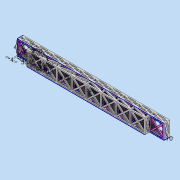
# Autodesk Inventor part: hashi1shado
Saved by Autodesk Inventor 2022 (Build 260153000, 153)
## iProperties
Created: 2024-05-14
Part Number: hashi1shado
Material: 一般
Document SubType Name: Modeling
Designer: ktamu
Density: 1 g/cm^3
Appearance: 既定
Mass: 103.699 g
Surface Area: 968.983 cm^2
Volume: 103.699 cm^3
Author: ktamu
Autodesk Inventor part; units mm, degrees
(part 1 of 2)
ref_plane "YZ Plane" through (0, 0, 0) normal (1, 0, 0) x (0, 1, 0)
ref_plane "XZ Plane" through (0, 0, 0) normal (0, 1, 0) x (-1, 0, 0)
ref_plane "XY Plane" through (0, 0, 0) normal (0, 0, 1) x (1, 0, 0)
sketch "スケッチ2" plane through (0, 0, 0) normal (1, 0, 0) x (0, 1, 0)
  line L0 (25, 10) -> (-25, 10)
  line L1 (-25, 10) -> (-25, -10)
  line L2 (-25, -10) -> (25, -10)
  line L3 (25, -10) -> (25, 10)
  line L4 (25, 10) -> (-25, -10) construction
  line L5 (-25, 10) -> (25, -10) construction
  point P0 (0, 0)
  dimension "d4" = 50
  dimension "d5" = 20
  constraints: 12 end point, 2 midpoint, 2 parallel, 1 horizontal, 1 perpendicular
  measures "d4" distance of L2.end L1.end
  measures "d5" distance of L1.end L0.end
sketch "スケッチ2 outline for 押し出し2" plane through (0, 0, 0) normal (1, 0, 0) x (0, 1, 0)
  line L0 (25, 10) -> (-25, 10)
  line L1 (25, -10) -> (25, 10)
  line L2 (-25, -10) -> (25, -10)
  line L3 (-25, 10) -> (-25, -10)
extrude "押し出し2" add sketch "スケッチ2 outline for 押し出し2" along normal mid plane 500
sketch "スケッチ3" plane through (-250, -25, 10) normal (0, 0, 1) x (1, 0, 0)
  circle A0 centre (250, 25) radius 5
  dimension "d8" = 10
  constraints: 1 centre point, 1 coincident
  measures "d8" diameter of A0
sketch "スケッチ3 outline for 押し出し3" plane through (-250, -25, 10) normal (0, 0, 1) x (1, 0, 0)
  circle A0 centre (250, 25) radius 5
extrude "押し出し3" add sketch "スケッチ3 outline for 押し出し3" along normal blind 2
sketch "SCfront" plane through (-250, -25, 10) normal (0, -1, 0) x (1, 0, 0)
  line L0 (0, -20) -> (500, -20)
  line L1 (500, 0) -> (500, -20)
  line L2 (500, 0) -> (0, 0)
  line L3 (0, -20) -> (0, 0)
  line L4 (0, 0) -> (500, 0)
  line L5 (500, 0) -> (500, -20)
  line L6 (500, -20) -> (0, -20)
  line L7 (0, -20) -> (0, 0)
  line L8 (0, 0) -> (500, -20) construction
  line L9 (500, 0) -> (0, -20) construction
  line L10 (0, 0) -> (500, 0)
  line L11 (0, -20) -> (500, -20)
  line L12 (0, 0) -> (50, 0)
  line L13 (50, 0) -> (50, -20)
  line L14 (50, -20) -> (0, -20)
  line L15 (0, -20) -> (0, 0)
  line L16 (100, 0) -> (100, -20)
  line L17 (150, 0) -> (150, -20)
  line L18 (200, 0) -> (200, -20)
  line L19 (250, 0) -> (250, -20)
  line L20 (450, 0) -> (450, -20)
  line L21 (400, 0) -> (400, -20)
  line L22 (350, 0) -> (350, -20)
  line L23 (300, 0) -> (300, -20)
  line L24 (0, 0) -> (0, -20)
  line L25 (0, 0) -> (50, -20)
  line L26 (0, -20) -> (50, 0) construction
  line L27 (50, 0) -> (100, -20)
  line L28 (100, 0) -> (50, -20)
  line L29 (52, -4) -> (98, -4)
  line L30 (98, -4) -> (98, -16)
  line L31 (98, -16) -> (52, -16)
  line L32 (52, -16) -> (52, -4)
  line L33 (75, -10) -> (98, -16) construction
  line L34 (98, -4) -> (52, -16) construction
  line L35 (102, -4) -> (148, -4)
  line L36 (102, -16) -> (102, -4)
  line L37 (148, -16) -> (102, -16)
  line L38 (148, -4) -> (148, -16)
  line L39 (152, -4) -> (198, -4)
  line L40 (152, -16) -> (152, -4)
  line L41 (198, -16) -> (152, -16)
  line L42 (198, -4) -> (198, -16)
  line L43 (202, -4) -> (248, -4)
  line L44 (202, -16) -> (202, -4)
  line L45 (248, -16) -> (202, -16)
  line L46 (248, -4) -> (248, -16)
  line L47 (252, -4) -> (298, -4)
  line L48 (252, -16) -> (252, -4)
  line L49 (298, -16) -> (252, -16)
  line L50 (298, -4) -> (298, -16)
  line L51 (302, -4) -> (348, -4)
  line L52 (302, -16) -> (302, -4)
  line L53 (348, -16) -> (302, -16)
  line L54 (348, -4) -> (348, -16)
  line L55 (352, -4) -> (398, -4)
  line L56 (352, -16) -> (352, -4)
  line L57 (398, -16) -> (352, -16)
  line L58 (398, -4) -> (398, -16)
  line L59 (402, -4) -> (448, -4)
  line L60 (402, -16) -> (402, -4)
  line L61 (448, -16) -> (402, -16)
  line L62 (448, -4) -> (448, -16)
  line L63 (48, -4) -> (48, -16)
  line L64 (48, -4) -> (4, -4)
  line L65 (4, -4) -> (4, -16.342138)
  line L66 (4, -16.342138) -> (48, -16.342138)
  line L67 (48, -16.342138) -> (48, -4)
  line L68 (452, -4) -> (452, -16)
  line L69 (452, -4) -> (496, -4)
  line L70 (496, -4) -> (496, -16.342138)
  line L71 (496, -16.342138) -> (452, -16.342138)
  line L72 (11.405237, -4) -> (48, -14.264946)
  line L73 (4, -6.077192) -> (40.594763, -16.342138)
  line L74 (488.594763, -4) -> (452, -14.264946)
  line L75 (496, -6.077192) -> (459.405237, -16.342138)
  line L76 (52, -4) -> (75, -10)
  line L77 (52, -6.066933) -> (90.076757, -16)
  line L78 (52.504844, -2.064765) -> (52.665247, -2.10661)
  line L79 (59.923243, -4) -> (98, -13.933067)
  line L80 (109.923243, -4) -> (148, -13.933067)
  line L81 (102, -6.066933) -> (140.076757, -16)
  line L82 (159.923243, -4) -> (198, -13.933067)
  line L83 (152, -6.066933) -> (190.076757, -16)
  line L84 (209.923243, -4) -> (248, -13.933067)
  line L85 (202, -6.066933) -> (240.076757, -16)
  line L86 (448, -6.066933) -> (409.923243, -16)
  line L87 (440.076757, -4) -> (402, -13.933067)
  line L88 (390.076757, -4) -> (352, -13.933067)
  line L89 (398, -6.066933) -> (359.923243, -16)
  line L90 (340.076757, -4) -> (302, -13.933067)
  line L91 (348, -6.066933) -> (309.923243, -16)
  line L92 (290.076757, -4) -> (252, -13.933067)
  line L93 (298, -6.066933) -> (259.923243, -16)
  line L94 (0, -10) -> (496, -10) construction
  line L95 (0, -10) -> (496, -10) construction
  line L96 (11.405237, -16) -> (48, -5.735054)
  line L97 (4, -13.922808) -> (39.375032, -4)
  line L98 (488.594763, -16) -> (452, -5.735054)
  line L99 (496, -13.922808) -> (459.405237, -3.657862)
  line L100 (52, -13.933067) -> (90.076757, -4)
  line L101 (59.923243, -16) -> (98, -6.066933)
  line L102 (109.923243, -16) -> (148, -6.066933)
  line L103 (102, -13.933067) -> (140.076757, -4)
  line L104 (159.923243, -16) -> (198, -6.066933)
  line L105 (152, -13.933067) -> (190.076757, -4)
  line L106 (209.923243, -16) -> (248, -6.066933)
  line L107 (202, -13.933067) -> (240.076757, -4)
  line L108 (448, -13.933067) -> (409.923243, -4)
  line L109 (440.076757, -16) -> (402, -6.066933)
  line L110 (398, -13.933067) -> (359.923243, -4)
  line L111 (390.076757, -16) -> (352, -6.066933)
  line L112 (348, -13.933067) -> (309.923243, -4)
  line L113 (340.076757, -16) -> (302, -6.066933)
  line L114 (298, -13.933067) -> (259.923243, -4)
  line L115 (290.076757, -16) -> (252, -6.066933)
  line L116 (25.390135, -12.077192) -> (10.185507, -16.342138)
  line L117 (474.609865, -12.077192) -> (489.814493, -16.342138)
  line L118 (50, 16) -> (50, -4)
  line L119 (100, 16) -> (100, -4)
  line L120 (150, 16) -> (150, -4)
  line L121 (250, 16) -> (250, -4)
  line L122 (450, 16) -> (450, -4)
  line L123 (300, 16) -> (300, -4)
  line L124 (350, 16) -> (350, -4)
  line L125 (400, 16) -> (400, -4)
  line L126 (200, 16) -> (200, -4)
  line L127 (152, 12) -> (198, 12)
  line L128 (198, 0) -> (152, 0)
  line L129 (152, 0) -> (152, 12)
  line L130 (148, 12) -> (148, 0)
  line L131 (109.923243, 12) -> (148, 2.066933)
  line L132 (148, 0) -> (102, 0)
  line L133 (102, 9.933067) -> (140.076757, 0)
  line L134 (102, 0) -> (102, 12)
  line L135 (50, 16) -> (100, -4)
  line L136 (100, 16) -> (50, -4)
  line L137 (102, 12) -> (148, 12)
  line L138 (52, 12) -> (98, 12)
  line L139 (98, 12) -> (98, 0)
  line L140 (98, 0) -> (52, 0)
  line L141 (52, 0) -> (52, 12)
  line L142 (75, 6) -> (98, 0) construction
  line L143 (98, 12) -> (52, 0) construction
  line L144 (198, 12) -> (198, 0)
  line L145 (202, 0) -> (202, 12)
  line L146 (248, 0) -> (202, 0)
  line L147 (248, 12) -> (248, 0)
  line L148 (202, 12) -> (248, 12)
  line L149 (252, 12) -> (298, 12)
  line L150 (59.923243, 12) -> (98, 2.066933)
  line L151 (59.923243, 0) -> (98, 9.933067)
  line L152 (52, 2.066933) -> (90.076757, 12)
  line L153 (52, 9.933067) -> (90.076757, 0)
  line L154 (352, 12) -> (398, 12)
  line L155 (352, 0) -> (352, 12)
  line L156 (398, 0) -> (352, 0)
  line L157 (398, 12) -> (398, 0)
  line L158 (402, 0) -> (402, 12)
  line L159 (402, 12) -> (448, 12)
  line L160 (448, 0) -> (402, 0)
  line L161 (448, 12) -> (448, 0)
  line L162 (52, 12) -> (75, 6)
  line L163 (252, 0) -> (252, 12)
  line L164 (298, 0) -> (252, 0)
  line L165 (298, 12) -> (298, 0)
  line L166 (302, 0) -> (302, 12)
  line L167 (302, 12) -> (348, 12)
  line L168 (348, 0) -> (302, 0)
  line L169 (348, 12) -> (348, 0)
  line L170 (52.504844, 13.935235) -> (52.665247, 13.89339)
  line L171 (209.923243, 12) -> (248, 2.066933)
  line L172 (202, 9.933067) -> (240.076757, 0)
  line L173 (209.923243, 0) -> (248, 9.933067)
  line L174 (202, 2.066933) -> (240.076757, 12)
  line L175 (448, 9.933067) -> (409.923243, 0)
  line L176 (440.076757, 12) -> (402, 2.066933)
  line L177 (448, 2.066933) -> (409.923243, 12)
  line L178 (440.076757, 0) -> (402, 9.933067)
  line L179 (290.076757, 12) -> (252, 2.066933)
  line L180 (290.076757, 0) -> (252, 9.933067)
  line L181 (298, 9.933067) -> (259.923243, 0)
  line L182 (298, 2.066933) -> (259.923243, 12)
  line L183 (340.076757, 12) -> (302, 2.066933)
  line L184 (340.076757, 0) -> (302, 9.933067)
  line L185 (348, 9.933067) -> (309.923243, 0)
  line L186 (348, 2.066933) -> (309.923243, 12)
  line L187 (398, 2.066933) -> (359.923243, 12)
  line L188 (390.076757, 12) -> (352, 2.066933)
  line L189 (390.076757, 0) -> (352, 9.933067)
  line L190 (398, 9.933067) -> (359.923243, 0)
  line L191 (102, 2.066933) -> (140.076757, 12)
  line L192 (109.923243, 0) -> (148, 9.933067)
  line L193 (152, 2.066933) -> (190.076757, 12)
  line L194 (159.923243, 12) -> (198, 2.066933)
  line L195 (159.923243, 0) -> (198, 9.933067)
  line L196 (152, 9.933067) -> (190.076757, 0)
  line L197 (50, 16) -> (450, 16)
  point P0 (250, -10)
  point P1 (440.076757, -4)
  point P2 (390.076757, -4)
  point P3 (340.076757, -4)
  point P4 (290.076757, -4)
  point P5 (209.923243, -4)
  point P6 (159.923243, -4)
  point P7 (109.923243, -4)
  point P8 (60.14392, -4.057568)
  point P9 (60, -4)
  point P10 (90, -16)
  point P11 (89.85608, -15.942432)
  point P12 (48, -14.264946)
  point P13 (40.594763, -3.657862)
  point P14 (482.015103, -10)
  point P15 (474.609865, -7.922808)
  point P16 (460.624968, -4)
  point P17 (467.204628, -10)
  point P18 (432.923243, -10)
  point P19 (425, -12.066933)
  point P20 (425, -7.933067)
  point P21 (417.076757, -10)
  point P22 (382.923243, -10)
  point P23 (375, -12.066933)
  point P24 (375, -7.933067)
  point P25 (367.076757, -10)
  point P26 (332.923243, -10)
  point P27 (325, -12.066933)
  point P28 (325, -7.933067)
  point P29 (317.076757, -10)
  point P30 (282.923243, -10)
  point P31 (275, -12.066933)
  point P32 (275, -7.933067)
  point P33 (267.076757, -10)
  point P34 (232.923243, -10)
  point P35 (225, -7.933067)
  point P36 (225, -12.066933)
  point P37 (217.076757, -10)
  point P38 (182.923243, -10)
  point P39 (175, -7.933067)
  point P40 (175, -12.066933)
  point P41 (167.076757, -10)
  point P42 (132.923243, -10)
  point P43 (125, -7.933067)
  point P44 (125, -12.066933)
  point P45 (117.076757, -10)
  point P46 (67.076757, -10)
  point P47 (59.923243, -16)
  point P48 (75, -12.066933)
  point P49 (75, -7.933067)
  point P50 (82.923243, -10)
  point P51 (25.390135, -7.922808)
  point P52 (32.795372, -10)
  point P53 (48, -5.735054)
  point P54 (11.405237, -16)
  point P55 (17.984897, -10)
  point P56 (4, -13.922808)
  point P57 (250, 6)
  point P58 (89.85608, 0.057568)
  point P59 (75, 3.933067)
  point P60 (60.14392, 0.057568)
  point P61 (60, 0)
  point P62 (90, 0)
  point P63 (67.076757, 6)
  point P64 (75, 8.066933)
  point P65 (89.85608, 11.942432)
  point P66 (90, 12)
  point P67 (60, 12)
  point P68 (60.14392, 11.942432)
  point P69 (82.923243, 6)
  point P70 (117.076757, 6)
  point P71 (125, 3.933067)
  point P72 (125, 8.066933)
  point P73 (109.923243, 12)
  point P74 (132.923243, 6)
  point P75 (148, 2.066933)
  point P76 (167.076757, 6)
  point P77 (159.923243, 12)
  point P78 (175, 8.066933)
  point P79 (175, 3.933067)
  point P80 (182.923243, 6)
  point P81 (198, 2.066933)
  point P82 (225, 3.933067)
  point P83 (217.076757, 6)
  point P84 (225, 8.066933)
  point P85 (209.923243, 12)
  point P86 (232.923243, 6)
  point P87 (248, 2.066933)
  point P88 (267.076757, 6)
  point P89 (252, 2.066933)
  point P90 (275, 3.933067)
  point P91 (275, 8.066933)
  point P92 (290.076757, 12)
  point P93 (282.923243, 6)
  point P94 (317.076757, 6)
  point P95 (302, 2.066933)
  point P96 (325, 3.933067)
  point P97 (325, 8.066933)
  point P98 (340.076757, 12)
  point P99 (332.923243, 6)
  point P100 (367.076757, 6)
  point P101 (352, 2.066933)
  point P102 (375, 8.066933)
  point P103 (390.076757, 12)
  point P104 (375, 3.933067)
  point P105 (382.923243, 6)
  point P106 (417.076757, 6)
  point P107 (402, 2.066933)
  point P108 (425, 3.933067)
  point P109 (425, 8.066933)
  point P110 (440.076757, 12)
  point P111 (432.923243, 6)
  point P112 (59.923243, 0)
  dimension "d12" = 50
  dimension "d15" = 50
  dimension "d20" = 46
  dimension "d21" = 12
  dimension "d24" = 50
  dimension "d29" = 4
  dimension "d30" = 4
  dimension "d33" = 4
  dimension "d37" = 2
  dimension "d40" = 50
  dimension "d96" = 0
  dimension "d97" = 10
  dimension "d106" = 16
  constraints: 382 end point, 73 symmetric about line, 28 horizontal alignment, 25 parallel, 25 point on line, 15 collinear, 8 midpoint, 7 horizontal, 5 perpendicular, 2 vertical, 228 other
  measures "d12" distance of L13.end L14.end
  measures "d15" distance of L12.end L16.start
  measures "d20" distance of L30.end L31.end
  measures "d21" distance of L29.end L30.end
  measures "d24" distance of L29.start L35.start
  measures "d29" distance between parallel lines of L32 L63
  measures "d30" distance between parallel lines of L65 L3
  measures "d33" distance between parallel lines of L12 L64
  measures "d37" distance between parallel lines of L76 L77
  measures "d40" distance of L79.start L80.start
  measures "d96" distance between parallel lines of L94 L95
  measures "d97" distance between parallel lines of L0 L95
  measures "d106" distance of L12.end L118.start
sketch "SCfront outline for 押し出し4" plane through (-250, -25, 10) normal (0, -1, 0) x (1, 0, 0)
  line L0 (496, -6.077192) -> (459.405237, -16.342138)
  line L1 (496, -16.342138) -> (496, -6.077192)
  line L2 (459.405237, -16.342138) -> (496, -16.342138)
  line L3 (452, -14.264946) -> (488.594763, -4)
  line L4 (452, -4) -> (452, -14.264946)
  line L5 (488.594763, -4) -> (452, -4)
  line L6 (448, -6.066933) -> (409.923243, -16)
  line L7 (448, -16) -> (448, -6.066933)
  line L8 (409.923243, -16) -> (448, -16)
  line L9 (402, -13.933067) -> (440.076757, -4)
  line L10 (402, -4) -> (402, -13.933067)
  line L11 (440.076757, -4) -> (402, -4)
  line L12 (398, -6.066933) -> (359.923243, -16)
  line L13 (398, -16) -> (398, -6.066933)
  line L14 (359.923243, -16) -> (398, -16)
  line L15 (352, -13.933067) -> (390.076757, -4)
  line L16 (352, -4) -> (352, -13.933067)
  line L17 (390.076757, -4) -> (352, -4)
  line L18 (348, -6.066933) -> (309.923243, -16)
  line L19 (348, -16) -> (348, -6.066933)
  line L20 (309.923243, -16) -> (348, -16)
  line L21 (302, -13.933067) -> (340.076757, -4)
  line L22 (302, -4) -> (302, -13.933067)
  line L23 (340.076757, -4) -> (302, -4)
  line L24 (298, -6.066933) -> (259.923243, -16)
  line L25 (298, -16) -> (298, -6.066933)
  line L26 (259.923243, -16) -> (298, -16)
  line L27 (252, -13.933067) -> (290.076757, -4)
  line L28 (252, -4) -> (252, -13.933067)
  line L29 (290.076757, -4) -> (252, -4)
  line L30 (209.923243, -4) -> (248, -13.933067)
  line L31 (248, -4) -> (209.923243, -4)
  line L32 (248, -13.933067) -> (248, -4)
  line L33 (240.076757, -16) -> (202, -6.066933)
  line L34 (202, -16) -> (240.076757, -16)
  line L35 (202, -6.066933) -> (202, -16)
  line L36 (159.923243, -4) -> (198, -13.933067)
  line L37 (198, -4) -> (159.923243, -4)
  line L38 (198, -13.933067) -> (198, -4)
  line L39 (190.076757, -16) -> (152, -6.066933)
  line L40 (152, -16) -> (190.076757, -16)
  line L41 (152, -6.066933) -> (152, -16)
  line L42 (109.923243, -4) -> (148, -13.933067)
  line L43 (148, -4) -> (109.923243, -4)
  line L44 (148, -13.933067) -> (148, -4)
  line L45 (140.076757, -16) -> (102, -6.066933)
  line L46 (102, -16) -> (140.076757, -16)
  line L47 (102, -6.066933) -> (102, -16)
  line L48 (60.14392, -4.057568) -> (98, -13.933067)
  line L49 (60, -4) -> (60.14392, -4.057568)
  line L50 (98, -4) -> (60, -4)
  line L51 (98, -13.933067) -> (98, -4)
  line L52 (89.85608, -15.942432) -> (52, -6.066933)
  line L53 (90, -16) -> (89.85608, -15.942432)
  line L54 (52, -16) -> (90, -16)
  line L55 (52, -6.066933) -> (52, -16)
  line L56 (11.405237, -4) -> (48, -14.264946)
  line L57 (48, -4) -> (11.405237, -4)
  line L58 (48, -14.264946) -> (48, -4)
  line L59 (40.594763, -16.342138) -> (4, -6.077192)
  line L60 (4, -16.342138) -> (40.594763, -16.342138)
  line L61 (4, -6.077192) -> (4, -16.342138)
extrude "押し出し4" cut sketch "SCfront outline for 押し出し4" against normal through all
sketch "SCLeft" plane through (-250, 0, 0) normal (-1, 0, 0) x (0, 0, 1)
  line L0 (10, 25) -> (10, -25)
  line L1 (-10, 25) -> (10, 25)
  line L2 (10, 25) -> (10, -25)
  line L3 (10, -25) -> (-10, -25)
  line L4 (-10, -25) -> (-10, 25)
  line L5 (-10, 25) -> (10, -25) construction
  line L6 (10, 25) -> (-10, -25) construction
  line L7 (-6, 21) -> (6, 21)
  line L8 (6, 21) -> (6, -21)
  line L9 (6, -21) -> (-6, -21)
  line L10 (-6, -21) -> (-6, 21)
  line L11 (-6, 21) -> (-1.040016, 3.640055) construction
  line L12 (6, 21) -> (-6, -21) construction
  line L13 (7.415352, 0) -> (4.34275, 0)
  line L14 (2.080031, 0) -> (6, -13.71989)
  line L15 (-3.919969, 21) -> (0, 7.28011)
  line L16 (-6, 21) -> (-1.040016, 3.640055)
  line L17 (1.040016, -3.640055) -> (6, -21)
  line L18 (-6, 13.71989) -> (-2.080031, 0)
  line L19 (0, -7.28011) -> (3.919969, -21)
  line L20 (0, 7.28011) -> (3.919969, 21)
  line L21 (-6, -13.71989) -> (-2.080031, 0)
  line L22 (-3.919969, -21) -> (0, -7.28011)
  line L23 (2.080031, 0) -> (6, 13.71989)
  point P0 (0, 0)
  dimension "d47" = 12
  dimension "d48" = 42
  constraints: 46 end point, 8 parallel, 5 point on line, 4 symmetric about line, 3 horizontal, 3 midpoint, 2 perpendicular
  measures "d47" distance of L8.end L9.end
  measures "d48" distance of L7.end L8.end
sketch "SCLeft outline for 押し出し5left" plane through (-250, 0, 0) normal (-1, 0, 0) x (0, 0, 1)
  line L0 (-6, 21) -> (-6, -21)
  line L1 (6, 21) -> (-6, 21)
  line L2 (6, -21) -> (6, 21)
  line L3 (-6, -21) -> (6, -21)
extrude "押し出し5left" cut sketch "SCLeft outline for 押し出し5left" against normal through all
sketch "SCLeft outline for 押し出し6" plane through (-250, 0, 0) normal (-1, 0, 0) x (0, 0, 1)
  line L0 (2.080031, 0) -> (6, 13.71989)
  line L1 (6, -13.71989) -> (2.080031, 0)
  line L2 (6, -21) -> (6, -13.71989)
  line L3 (3.919969, -21) -> (6, -21)
  line L4 (0, -7.28011) -> (3.919969, -21)
  line L5 (-3.919969, -21) -> (0, -7.28011)
  line L6 (-6, -21) -> (-3.919969, -21)
  line L7 (-6, -13.71989) -> (-6, -21)
  line L8 (-2.080031, 0) -> (-6, -13.71989)
  line L9 (-6, 13.71989) -> (-2.080031, 0)
  line L10 (-6, 21) -> (-6, 13.71989)
  line L11 (-3.919969, 21) -> (-6, 21)
  line L12 (0, 7.28011) -> (-3.919969, 21)
  line L13 (3.919969, 21) -> (0, 7.28011)
  line L14 (6, 21) -> (3.919969, 21)
  line L15 (6, 13.71989) -> (6, 21)
extrude "押し出し6" add sketch "SCLeft outline for 押し出し6" against normal blind 4
mirror "ミラー1" about plane through (0, 0, 0) normal (1, 0, 0) of "押し出し6"
sketch "SCtop" plane through (-250, -25, 10) normal (0, 0, 1) x (1, 0, 0)
  circle A0 centre (250, 25) radius 5
  line L0 (500, 0) -> (0, 0)
  line L1 (500, 50) -> (500, 0)
  line L2 (0, 50) -> (500, 50)
  line L3 (0, 0) -> (0, 50)
  circle A1 centre (250, 25) radius 5
  line L4 (0, 0) -> (0, 50)
  line L5 (0, 50) -> (500, 0) construction
  line L6 (0, 0) -> (500, 0)
  line L7 (500, 50) -> (0, 0) construction
  line L8 (0, 50) -> (500, 50)
  line L9 (500, 50) -> (500, 0)
  line L10 (500, 0) -> (0, 0)
  line L11 (0, 0) -> (0, 50)
  line L12 (0, 50) -> (500, 0) construction
  line L13 (500, 50) -> (0, 0) construction
  line L14 (0, 50) -> (500, 50)
  line L15 (0, 50) -> (50, 50)
  line L16 (50, 50) -> (50, 0)
  line L17 (50, 0) -> (0, 0)
  line L18 (0, 0) -> (0, 50)
  line L19 (100, 50) -> (100, 0)
  line L20 (150, 50) -> (150, 0)
  line L21 (200, 50) -> (200, 0)
  line L22 (250, 50) -> (250, 0)
  line L23 (300, 50) -> (300, 0)
  line L24 (350, 50) -> (350, 0)
  line L25 (400, 50) -> (400, 0)
  line L26 (450, 50) -> (450, 0)
  line L27 (50, 50) -> (100, 0)
  line L28 (0, 50) -> (50, 0)
  line L29 (50, 50) -> (0, 0)
  line L30 (98, 4) -> (60.14392, 4)
  line L31 (52, 46) -> (98, 46)
  line L32 (98, 46) -> (98, 4)
  line L33 (98, 4) -> (52, 4)
  line L34 (52, 4) -> (52, 46)
  line L35 (4, 46) -> (48, 46)
  line L36 (48, 46) -> (48, 4)
  line L37 (48, 4) -> (4, 4)
  line L38 (4, 4) -> (4, 46)
  line L39 (6.828427, 46) -> (48.025843, 4.802584)
  line L40 (4, 43.171573) -> (43.171573, 4)
  line L41 (25, 25) -> (25, 18.621886)
  line L42 (98, 0) -> (98, 4)
  line L43 (53.475936, 44.652406) -> (98, 4)
  line L44 (52, 43.291755) -> (95.033826, 4)
  line L45 (54.966174, 46) -> (98, 6.708245)
  line L46 (98, 43.291755) -> (54.966174, 4)
  line L47 (92.274678, 40.772532) -> (53.475936, 5.347594)
  line L48 (95.033826, 46) -> (52, 6.708245)
  line L49 (50.144939, 5.014494) -> (50, 4.882159)
  line L50 (73.584326, 23.584326) -> (90.909091, 40.909091)
  line L51 (92.274678, 40.772532) -> (73.516913, 23.645877) construction
  line L52 (53.475936, 5.347594) -> (52, 4) construction
  line L53 (52, 46) -> (53.475936, 44.652406) construction
  line L54 (73.516913, 26.354123) -> (98, 4) construction
  line L55 (48, 46) -> (4, 4)
  line L56 (45.103446, 46) -> (4, 6.764892)
  line L57 (48, 43.235108) -> (6.896554, 4)
  line L58 (104.966174, 46) -> (148, 6.708245)
  line L59 (145.033826, 46) -> (102, 6.708245)
  line L60 (148, 43.291755) -> (104.966174, 4)
  line L61 (102, 43.291755) -> (145.033826, 4)
  line L62 (148, 46) -> (148, 4)
  line L63 (102, 46) -> (148, 46)
  line L64 (102, 4) -> (102, 46)
  line L65 (148, 4) -> (102, 4)
  line L66 (154.966174, 46) -> (198, 6.708245)
  line L67 (195.033826, 46) -> (152, 6.708245)
  line L68 (198, 43.291755) -> (154.966174, 4)
  line L69 (152, 43.291755) -> (195.033826, 4)
  line L70 (198, 46) -> (198, 4)
  line L71 (152, 46) -> (198, 46)
  line L72 (152, 4) -> (152, 46)
  line L73 (198, 4) -> (152, 4)
  line L74 (204.966174, 46) -> (248, 6.708245)
  line L75 (245.033826, 46) -> (202, 6.708245)
  line L76 (248, 43.291755) -> (204.966174, 4)
  line L77 (202, 43.291755) -> (245.033826, 4)
  line L78 (248, 46) -> (248, 4)
  line L79 (202, 46) -> (248, 46)
  line L80 (202, 4) -> (202, 46)
  line L81 (248, 4) -> (202, 4)
  line L82 (254.966174, 46) -> (298, 6.708245)
  line L83 (295.033826, 46) -> (252, 6.708245)
  line L84 (298, 43.291755) -> (254.966174, 4)
  line L85 (252, 43.291755) -> (295.033826, 4)
  line L86 (298, 46) -> (298, 4)
  line L87 (252, 46) -> (298, 46)
  line L88 (252, 4) -> (252, 46)
  line L89 (298, 4) -> (252, 4)
  line L90 (304.966174, 46) -> (348, 6.708245)
  line L91 (345.033826, 46) -> (302, 6.708245)
  line L92 (348, 43.291755) -> (304.966174, 4)
  line L93 (302, 43.291755) -> (345.033826, 4)
  line L94 (348, 46) -> (348, 4)
  line L95 (302, 46) -> (348, 46)
  line L96 (302, 4) -> (302, 46)
  line L97 (348, 4) -> (302, 4)
  line L98 (354.966174, 46) -> (398, 6.708245)
  line L99 (395.033826, 46) -> (352, 6.708245)
  line L100 (398, 43.291755) -> (354.966174, 4)
  line L101 (352, 43.291755) -> (395.033826, 4)
  line L102 (398, 46) -> (398, 4)
  line L103 (352, 46) -> (398, 46)
  line L104 (352, 4) -> (352, 46)
  line L105 (398, 4) -> (352, 4)
  line L106 (404.966174, 46) -> (448, 6.708245)
  line L107 (445.033826, 46) -> (402, 6.708245)
  line L108 (448, 43.291755) -> (404.966174, 4)
  line L109 (402, 43.291755) -> (445.033826, 4)
  line L110 (448, 46) -> (448, 4)
  line L111 (402, 46) -> (448, 46)
  line L112 (402, 4) -> (402, 46)
  line L113 (448, 4) -> (402, 4)
  line L114 (496, 46) -> (452, 46)
  line L115 (452, 46) -> (452, 4)
  line L116 (452, 4) -> (496, 4)
  line L117 (496, 4) -> (496, 46)
  line L118 (493.171573, 46) -> (451.974157, 4.802584)
  line L119 (496, 43.171573) -> (456.828427, 4)
  line L120 (454.896554, 46) -> (496, 6.764892)
  line L121 (452, 43.235108) -> (493.103446, 4)
  point P0 (75, 25)
  point P1 (123.516913, 26.354123)
  point P2 (123.584326, 23.584326)
  point P3 (123.516913, 23.645877)
  point P4 (173.516913, 26.354123)
  point P5 (173.584326, 23.584326)
  point P6 (173.516913, 23.645877)
  point P7 (223.516913, 26.354123)
  point P8 (223.584326, 23.584326)
  point P9 (223.516913, 23.645877)
  point P10 (273.516913, 26.354123)
  point P11 (273.584326, 23.584326)
  point P12 (273.516913, 23.645877)
  point P13 (323.516913, 26.354123)
  point P14 (323.584326, 23.584326)
  point P15 (323.516913, 23.645877)
  point P16 (373.516913, 26.354123)
  point P17 (373.584326, 23.584326)
  point P18 (373.516913, 23.645877)
  point P19 (423.516913, 26.354123)
  point P20 (423.584326, 23.584326)
  point P21 (423.516913, 23.645877)
  point P22 (474.544134, 21.715707)
  point P23 (477.373326, 24.544899)
  point P24 (474.479122, 27.307549)
  point P25 (452, 4.828427)
  point P26 (471.64993, 24.478357)
  point P27 (427.966174, 25)
  point P28 (425, 22.291755)
  point P29 (425, 27.708245)
  point P30 (375, 22.291755)
  point P31 (375, 27.708245)
  point P32 (422.033826, 25)
  point P33 (377.966174, 25)
  point P34 (372.033826, 25)
  point P35 (327.966174, 25)
  point P36 (325, 22.291755)
  point P37 (325, 27.708245)
  point P38 (322.033826, 25)
  point P39 (275, 22.291755)
  point P40 (277.966174, 25)
  point P41 (275, 27.708245)
  point P42 (252, 20.417424)
  point P43 (272.033826, 25)
  point P44 (252, 29.582576)
  point P45 (225, 22.291755)
  point P46 (248, 29.582576)
  point P47 (227.966174, 25)
  point P48 (248, 20.417424)
  point P49 (225, 27.708245)
  point P50 (222.033826, 25)
  point P51 (175, 22.291755)
  point P52 (177.966174, 25)
  point P53 (175, 27.708245)
  point P54 (172.033826, 25)
  point P55 (125, 22.291755)
  point P56 (127.966174, 25)
  point P57 (125, 27.708245)
  point P58 (122.033826, 25)
  point P59 (77.966174, 25)
  point P60 (75, 22.291755)
  point P61 (75, 27.708245)
  point P62 (72.033826, 25)
  point P63 (25.455866, 21.715707)
  point P64 (28.35007, 24.478357)
  point P65 (48, 4.828427)
  point P66 (22.626674, 24.544899)
  point P67 (25.520878, 27.307549)
  dimension "d55" = 50
  dimension "d56" = 50
  dimension "d59" = 50
  dimension "d64" = 46
  dimension "d65" = 42
  dimension "d66" = 44
  dimension "d67" = 42
  dimension "d68" = 4
  dimension "d69" = 4
  dimension "d76" = 2
  dimension "d77" = 2
  dimension "d80" = 50
  constraints: 226 end point, 97 point on line, 20 midpoint, 17 parallel, 12 symmetric about line, 6 horizontal, 5 perpendicular, 1 vertical, 185 other
  measures "d55" distance of L16.end L17.end
  measures "d56" distance of L15.end L16.end
  measures "d59" distance of L15.end L19.start
  measures "d64" distance of L30.start L33.end
  measures "d65" distance of L31.end L30.start
  measures "d66" distance of L36.end L37.end
  measures "d67" distance of L35.end L36.end
  measures "d68" distance between parallel lines of L2 L35
  measures "d69" distance between parallel lines of L34 L36
  measures "d76" distance between parallel lines of L55 L56
  measures "d77" distance between parallel lines of L55 L57
  measures "d80" distance of L45.start L58.start
sketch "SCtop outline for 押し出し7" plane through (-250, -25, 10) normal (0, 0, 1) x (1, 0, 0)
  line L0 (456.828427, 4) -> (493.103446, 4)
  line L1 (474.544134, 21.715707) -> (456.828427, 4)
  line L2 (493.103446, 4) -> (474.544134, 21.715707)
  line L3 (496, 6.764892) -> (496, 43.171573)
  line L4 (477.373326, 24.544899) -> (496, 6.764892)
  line L5 (496, 43.171573) -> (477.373326, 24.544899)
  line L6 (493.171573, 46) -> (454.896554, 46)
  line L7 (474.479122, 27.307549) -> (493.171573, 46)
  line L8 (454.896554, 46) -> (474.479122, 27.307549)
  line L9 (452, 43.235108) -> (452, 4.828427)
  line L10 (471.64993, 24.478357) -> (452, 43.235108)
  line L11 (452, 4.828427) -> (471.64993, 24.478357)
  line L12 (448, 6.708245) -> (448, 43.291755)
  line L13 (427.966174, 25) -> (448, 6.708245)
  line L14 (448, 43.291755) -> (427.966174, 25)
  line L15 (404.966174, 4) -> (445.033826, 4)
  line L16 (425, 22.291755) -> (404.966174, 4)
  line L17 (445.033826, 4) -> (425, 22.291755)
  line L18 (445.033826, 46) -> (404.966174, 46)
  line L19 (425, 27.708245) -> (445.033826, 46)
  line L20 (404.966174, 46) -> (425, 27.708245)
  line L21 (354.966174, 4) -> (395.033826, 4)
  line L22 (375, 22.291755) -> (354.966174, 4)
  line L23 (395.033826, 4) -> (375, 22.291755)
  line L24 (395.033826, 46) -> (354.966174, 46)
  line L25 (375, 27.708245) -> (395.033826, 46)
  line L26 (354.966174, 46) -> (375, 27.708245)
  line L27 (402, 43.291755) -> (402, 6.708245)
  line L28 (422.033826, 25) -> (402, 43.291755)
  line L29 (402, 6.708245) -> (422.033826, 25)
  line L30 (398, 6.708245) -> (398, 43.291755)
  line L31 (377.966174, 25) -> (398, 6.708245)
  line L32 (398, 43.291755) -> (377.966174, 25)
  line L33 (352, 43.291755) -> (352, 6.708245)
  line L34 (372.033826, 25) -> (352, 43.291755)
  line L35 (352, 6.708245) -> (372.033826, 25)
  line L36 (348, 6.708245) -> (348, 43.291755)
  line L37 (327.966174, 25) -> (348, 6.708245)
  line L38 (348, 43.291755) -> (327.966174, 25)
  line L39 (304.966174, 4) -> (345.033826, 4)
  line L40 (325, 22.291755) -> (304.966174, 4)
  line L41 (345.033826, 4) -> (325, 22.291755)
  line L42 (345.033826, 46) -> (304.966174, 46)
  line L43 (325, 27.708245) -> (345.033826, 46)
  line L44 (304.966174, 46) -> (325, 27.708245)
  line L45 (302, 43.291755) -> (302, 6.708245)
  line L46 (322.033826, 25) -> (302, 43.291755)
  line L47 (302, 6.708245) -> (322.033826, 25)
  line L48 (254.966174, 4) -> (295.033826, 4)
  line L49 (275, 22.291755) -> (254.966174, 4)
  line L50 (295.033826, 4) -> (275, 22.291755)
  line L51 (298, 6.708245) -> (298, 43.291755)
  line L52 (277.966174, 25) -> (298, 6.708245)
  line L53 (298, 43.291755) -> (277.966174, 25)
  line L54 (295.033826, 46) -> (254.966174, 46)
  line L55 (275, 27.708245) -> (295.033826, 46)
  line L56 (254.966174, 46) -> (275, 27.708245)
  line L57 (252, 20.417424) -> (252, 6.708245)
  arc A0 (252, 29.582576) -> (252, 20.417424) centre (250, 25) cw
  line L58 (252, 43.291755) -> (252, 29.582576)
  line L59 (272.033826, 25) -> (252, 43.291755)
  line L60 (252, 6.708245) -> (272.033826, 25)
  line L61 (204.966174, 4) -> (245.033826, 4)
  line L62 (225, 22.291755) -> (204.966174, 4)
  line L63 (245.033826, 4) -> (225, 22.291755)
  line L64 (248, 29.582576) -> (248, 43.291755)
  arc A1 (248, 20.417424) -> (248, 29.582576) centre (250, 25) cw
  line L65 (248, 6.708245) -> (248, 20.417424)
  line L66 (227.966174, 25) -> (248, 6.708245)
  line L67 (248, 43.291755) -> (227.966174, 25)
  line L68 (245.033826, 46) -> (204.966174, 46)
  line L69 (225, 27.708245) -> (245.033826, 46)
  line L70 (204.966174, 46) -> (225, 27.708245)
  line L71 (202, 43.291755) -> (202, 6.708245)
  line L72 (222.033826, 25) -> (202, 43.291755)
  line L73 (202, 6.708245) -> (222.033826, 25)
  line L74 (154.966174, 4) -> (195.033826, 4)
  line L75 (175, 22.291755) -> (154.966174, 4)
  line L76 (195.033826, 4) -> (175, 22.291755)
  line L77 (198, 6.708245) -> (198, 43.291755)
  line L78 (177.966174, 25) -> (198, 6.708245)
  line L79 (198, 43.291755) -> (177.966174, 25)
  line L80 (195.033826, 46) -> (154.966174, 46)
  line L81 (175, 27.708245) -> (195.033826, 46)
  line L82 (154.966174, 46) -> (175, 27.708245)
  line L83 (152, 43.291755) -> (152, 6.708245)
  line L84 (172.033826, 25) -> (152, 43.291755)
  line L85 (152, 6.708245) -> (172.033826, 25)
  line L86 (104.966174, 4) -> (145.033826, 4)
  line L87 (125, 22.291755) -> (104.966174, 4)
  line L88 (145.033826, 4) -> (125, 22.291755)
  line L89 (148, 6.708245) -> (148, 43.291755)
  line L90 (127.966174, 25) -> (148, 6.708245)
  line L91 (148, 43.291755) -> (127.966174, 25)
  line L92 (145.033826, 46) -> (104.966174, 46)
  line L93 (125, 27.708245) -> (145.033826, 46)
  line L94 (104.966174, 46) -> (125, 27.708245)
  line L95 (102, 43.291755) -> (102, 6.708245)
  line L96 (122.033826, 25) -> (102, 43.291755)
  line L97 (102, 6.708245) -> (122.033826, 25)
  line L98 (98, 43.291755) -> (77.966174, 25)
  line L99 (98, 6.708245) -> (98, 43.291755)
  line L100 (77.966174, 25) -> (98, 6.708245)
  line L101 (75, 22.291755) -> (54.966174, 4)
  line L102 (54.966174, 4) -> (95.033826, 4)
  line L103 (95.033826, 4) -> (75, 22.291755)
  line L104 (75, 27.708245) -> (95.033826, 46)
  line L105 (54.966174, 46) -> (75, 27.708245)
  line L106 (95.033826, 46) -> (54.966174, 46)
  line L107 (52, 6.708245) -> (72.033826, 25)
  line L108 (52, 43.291755) -> (52, 6.708245)
  line L109 (72.033826, 25) -> (52, 43.291755)
  line L110 (25.455866, 21.715707) -> (6.896554, 4)
  line L111 (43.171573, 4) -> (25.455866, 21.715707)
  line L112 (6.896554, 4) -> (43.171573, 4)
  line L113 (48, 43.235108) -> (28.35007, 24.478357)
  line L114 (48, 4.828427) -> (48, 43.235108)
  line L115 (28.35007, 24.478357) -> (48, 4.828427)
  line L116 (4, 6.764892) -> (22.626674, 24.544899)
  line L117 (4, 43.171573) -> (4, 6.764892)
  line L118 (22.626674, 24.544899) -> (4, 43.171573)
  line L119 (25.520878, 27.307549) -> (45.103446, 46)
  line L120 (6.828427, 46) -> (25.520878, 27.307549)
  line L121 (45.103446, 46) -> (6.828427, 46)
extrude "押し出し7" cut sketch "SCtop outline for 押し出し7" against normal through all
sketch "スケッチ7" plane through (0, 0, 12) normal (0, 0, 1) x (1, 0, 0)
  line L0 (-2, 21) -> (-2, -21)
  line L1 (2, -18.291755) -> (2, -4.582576)
  line L2 (2, -21) -> (2, 21)
  circle A0 centre (0, 0) radius 5
  arc A1 (-2, -4.582576) -> (2, -4.582576) centre (0, 0) ccw
  line L3 (-2, -4.582576) -> (-2, 4.582576)
  line L4 (2, -4.582576) -> (2, 4.582576)
  circle A2 centre (0, 0) radius 1
  point P0 (-2, -4.582576)
  dimension "d89" = 2
  constraints: 4 end point, 2 point on circle, 2 point on line, 1 centre point, 1 coincident
  measures "d89" diameter of A2
sketch "スケッチ7 outline for 押し出し8" plane through (0, 0, 12) normal (0, 0, 1) x (1, 0, 0)
  arc A0 (2, -4.582576) -> (2, 4.582576) centre (0, 0) ccw
  line L0 (2, 4.582576) -> (2, -4.582576)
  arc A1 (-2, 4.582576) -> (-2, -4.582576) centre (0, 0) ccw
  line L1 (-2, -4.582576) -> (-2, 4.582576)
extrude "押し出し8" cut sketch "スケッチ7 outline for 押し出し8" against normal through all
sketch "スケッチ7 outline for 押し出し9" plane through (0, 0, 12) normal (0, 0, 1) x (1, 0, 0)
  arc A0 (-2, -4.582576) -> (2, -4.582576) centre (0, 0) ccw
  line L0 (-2, 4.582576) -> (-2, -4.582576)
  line L1 (2, -4.582576) -> (2, 4.582576)
  arc A1 (2, 4.582576) -> (-2, 4.582576) centre (0, 0) ccw
  circle A2 centre (0, 0) radius 1
extrude "押し出し9" cut sketch "スケッチ7 outline for 押し出し9" against normal blind 2
sketch "スケッチ7 outline for 押し出し10" plane through (0, 0, 12) normal (0, 0, 1) x (1, 0, 0)
  circle A0 centre (0, 0) radius 1
extrude "押し出し10" cut sketch "スケッチ7 outline for 押し出し10" against normal blind 1
sketch "スケッチ7 outline for 押し出し11" plane through (0, 0, 12) normal (0, 0, 1) x (1, 0, 0)
  circle A0 centre (0, 0) radius 1
extrude "押し出し11" cut sketch "スケッチ7 outline for 押し出し11" against normal blind 2
sketch "SCfront outline for 押し出し12" plane through (-250, -25, 10) normal (0, -1, 0) x (1, 0, 0)
  line L0 (496, -13.922808) -> (482.015103, -10)
  line L1 (496, -16.342138) -> (496, -13.922808)
  line L2 (459.405237, -16.342138) -> (496, -16.342138)
  line L3 (482.015103, -10) -> (459.405237, -16.342138)
  line L4 (474.609865, -7.922808) -> (460.624968, -4)
  line L5 (467.204628, -10) -> (474.609865, -7.922808)
  line L6 (452, -5.735054) -> (467.204628, -10)
  line L7 (452, -4) -> (452, -5.735054)
  line L8 (460.624968, -4) -> (452, -4)
  line L9 (448, -13.933067) -> (432.923243, -10)
  line L10 (448, -16) -> (448, -13.933067)
  line L11 (440.076757, -16) -> (448, -16)
  line L12 (425, -12.066933) -> (440.076757, -16)
  line L13 (432.923243, -10) -> (425, -12.066933)
  line L14 (425, -7.933067) -> (409.923243, -4)
  line L15 (417.076757, -10) -> (425, -7.933067)
  line L16 (402, -6.066933) -> (417.076757, -10)
  line L17 (402, -4) -> (402, -6.066933)
  line L18 (409.923243, -4) -> (402, -4)
  line L19 (398, -13.933067) -> (382.923243, -10)
  line L20 (398, -16) -> (398, -13.933067)
  line L21 (390.076757, -16) -> (398, -16)
  line L22 (375, -12.066933) -> (390.076757, -16)
  line L23 (382.923243, -10) -> (375, -12.066933)
  line L24 (375, -7.933067) -> (359.923243, -4)
  line L25 (367.076757, -10) -> (375, -7.933067)
  line L26 (352, -6.066933) -> (367.076757, -10)
  line L27 (352, -4) -> (352, -6.066933)
  line L28 (359.923243, -4) -> (352, -4)
  line L29 (348, -13.933067) -> (332.923243, -10)
  line L30 (348, -16) -> (348, -13.933067)
  line L31 (340.076757, -16) -> (348, -16)
  line L32 (325, -12.066933) -> (340.076757, -16)
  line L33 (332.923243, -10) -> (325, -12.066933)
  line L34 (325, -7.933067) -> (309.923243, -4)
  line L35 (317.076757, -10) -> (325, -7.933067)
  line L36 (302, -6.066933) -> (317.076757, -10)
  line L37 (302, -4) -> (302, -6.066933)
  line L38 (309.923243, -4) -> (302, -4)
  line L39 (298, -13.933067) -> (282.923243, -10)
  line L40 (298, -16) -> (298, -13.933067)
  line L41 (290.076757, -16) -> (298, -16)
  line L42 (275, -12.066933) -> (290.076757, -16)
  line L43 (282.923243, -10) -> (275, -12.066933)
  line L44 (275, -7.933067) -> (259.923243, -4)
  line L45 (267.076757, -10) -> (275, -7.933067)
  line L46 (252, -6.066933) -> (267.076757, -10)
  line L47 (252, -4) -> (252, -6.066933)
  line L48 (259.923243, -4) -> (252, -4)
  line L49 (232.923243, -10) -> (248, -6.066933)
  line L50 (225, -7.933067) -> (232.923243, -10)
  line L51 (240.076757, -4) -> (225, -7.933067)
  line L52 (248, -4) -> (240.076757, -4)
  line L53 (248, -6.066933) -> (248, -4)
  line L54 (209.923243, -16) -> (225, -12.066933)
  line L55 (202, -16) -> (209.923243, -16)
  line L56 (202, -13.933067) -> (202, -16)
  line L57 (217.076757, -10) -> (202, -13.933067)
  line L58 (225, -12.066933) -> (217.076757, -10)
  line L59 (182.923243, -10) -> (198, -6.066933)
  line L60 (175, -7.933067) -> (182.923243, -10)
  line L61 (190.076757, -4) -> (175, -7.933067)
  line L62 (198, -4) -> (190.076757, -4)
  line L63 (198, -6.066933) -> (198, -4)
  line L64 (159.923243, -16) -> (175, -12.066933)
  line L65 (152, -16) -> (159.923243, -16)
  line L66 (152, -13.933067) -> (152, -16)
  line L67 (167.076757, -10) -> (152, -13.933067)
  line L68 (175, -12.066933) -> (167.076757, -10)
  line L69 (132.923243, -10) -> (148, -6.066933)
  line L70 (125, -7.933067) -> (132.923243, -10)
  line L71 (140.076757, -4) -> (125, -7.933067)
  line L72 (148, -4) -> (140.076757, -4)
  line L73 (148, -6.066933) -> (148, -4)
  line L74 (109.923243, -16) -> (125, -12.066933)
  line L75 (102, -16) -> (109.923243, -16)
  line L76 (102, -13.933067) -> (102, -16)
  line L77 (117.076757, -10) -> (102, -13.933067)
  line L78 (125, -12.066933) -> (117.076757, -10)
  line L79 (67.076757, -10) -> (52, -13.933067)
  line L80 (75, -12.066933) -> (67.076757, -10)
  line L81 (59.923243, -16) -> (75, -12.066933)
  line L82 (52, -16) -> (59.923243, -16)
  line L83 (52, -13.933067) -> (52, -16)
  line L84 (90.076757, -4) -> (75, -7.933067)
  line L85 (98, -4) -> (90.076757, -4)
  line L86 (98, -6.066933) -> (98, -4)
  line L87 (82.923243, -10) -> (98, -6.066933)
  line L88 (75, -7.933067) -> (82.923243, -10)
  line L89 (39.375032, -4) -> (25.390135, -7.922808)
  line L90 (48, -4) -> (39.375032, -4)
  line L91 (48, -5.735054) -> (48, -4)
  line L92 (32.795372, -10) -> (48, -5.735054)
  line L93 (25.390135, -7.922808) -> (32.795372, -10)
  line L94 (10.185507, -16.342138) -> (25.390135, -12.077192)
  line L95 (25.390135, -12.077192) -> (17.984897, -10)
  line L96 (17.984897, -10) -> (4, -13.922808)
  line L97 (4, -13.922808) -> (4, -16.342138)
  line L98 (4, -16.342138) -> (10.185507, -16.342138)
extrude "押し出し12" add sketch "SCfront outline for 押し出し12" against normal blind 4
sketch "SCfront outline for 押し出し13" plane through (-250, -25, 10) normal (0, -1, 0) x (1, 0, 0)
  line L0 (489.814493, -16.342138) -> (488.594763, -16)
  line L1 (459.405237, -16.342138) -> (489.814493, -16.342138)
  line L2 (474.609865, -12.077192) -> (459.405237, -16.342138)
  line L3 (488.594763, -16) -> (474.609865, -12.077192)
extrude "押し出し13" cut sketch "SCfront outline for 押し出し13" against normal blind 88.5
mirror "ミラー2" about plane through (0, 0, 0) normal (0, 1, 0) of "押し出し12"
sketch "SCfront outline for 押し出し14" plane through (-250, -25, 10) normal (0, -1, 0) x (1, 0, 0)
  line L0 (489.814493, -16.342138) -> (488.594763, -16)
  line L1 (459.405237, -16.342138) -> (489.814493, -16.342138)
  line L2 (474.609865, -12.077192) -> (459.405237, -16.342138)
  line L3 (488.594763, -16) -> (474.609865, -12.077192)
extrude "押し出し14" cut sketch "SCfront outline for 押し出し14" against normal blind 84
sketch "スケッチ8" plane through (0, 0, 0) normal (0, 0, 1) x (1, 0, 0)
  point P0 (0, 0)
sketch "スケッチ9" plane through (0, 0, 0) normal (1, 0, 0) x (0, 1, 0)
  line L0 (25, 10) -> (25, -10) projected
  line L1 (25, 10) -> (-25, 10)
  line L2 (-25, 10) -> (-25, 26)
  line L3 (-25, 26) -> (25, 26)
  line L4 (25, 26) -> (25, 10)
  point P0 (0, 0)
  dimension "d111" = 50
  dimension "d112" = 16
  constraints: 8 end point, 2 parallel, 1 horizontal, 1 perpendicular
  measures "d111" distance of L2.end L3.end
  measures "d112" distance of L1.end L2.end
sketch "スケッチ9 outline for 押し出し15" plane through (0, 0, 0) normal (1, 0, 0) x (0, 1, 0)
  line L0 (25, 10) -> (25, 26)
  line L1 (-25, 10) -> (25, 10)
  line L2 (-25, 26) -> (-25, 10)
  line L3 (25, 26) -> (-25, 26)
extrude "押し出し15" add sketch "スケッチ9 outline for 押し出し15" along normal mid plane 404
sketch "スケッチ10" plane through (202, 18.235108, 10) normal (1, 0, 0) x (0, 0, -1)
  line L0 (0, 2.764892) -> (-12, 2.764892)
  line L1 (-12, 2.764892) -> (-12, -39.235108)
  line L2 (-12, -39.235108) -> (0, -39.235108)
  line L3 (0, -39.235108) -> (0, 2.764892)
  line L4 (0, 6.764892) -> (-16, 6.764892)
  line L5 (-16, 6.764892) -> (-16, -43.235108)
  line L6 (-16, -43.235108) -> (0, -43.235108)
  line L7 (0, 6.764892) -> (0, -43.235108)
  point P0 (10, -18.235108)
  dimension "d115" = 4
  dimension "d116" = 4
  dimension "d117" = 4
  dimension "d118" = 0
  constraints: 8 end point, 2 parallel, 1 horizontal, 1 perpendicular
  measures "d115" distance between parallel lines of L4 L0
  measures "d116" distance between parallel lines of L1 L5
  measures "d117" distance between parallel lines of L6 L2
  measures "d118" distance between parallel lines of L7 L3
sketch "スケッチ10 outline for 押し出し16" plane through (202, 18.235108, 10) normal (1, 0, 0) x (0, 0, -1)
  line L0 (-12, 2.764892) -> (-12, -39.235108)
  line L1 (0, 2.764892) -> (-12, 2.764892)
  line L2 (0, -39.235108) -> (0, 2.764892)
  line L3 (-12, -39.235108) -> (0, -39.235108)
extrude "押し出し16" cut sketch "スケッチ10 outline for 押し出し16" against normal through all
sketch "SCfront outline for 押し出し17" plane through (-250, -25, 10) normal (0, -1, 0) x (1, 0, 0)
  line L0 (89.85608, 0.057568) -> (52, 9.933067)
  line L1 (52, 9.933067) -> (52, 0)
  line L2 (52, 0) -> (59.923243, 0)
  line L3 (59.923243, 0) -> (60.14392, 0.057568)
  line L4 (60.14392, 0.057568) -> (60, 0)
  line L5 (60, 0) -> (90, 0)
  line L6 (90, 0) -> (89.85608, 0.057568)
  line L7 (60.14392, 11.942432) -> (98, 2.066933)
  line L8 (98, 2.066933) -> (98, 12)
  line L9 (98, 12) -> (90.076757, 12)
  line L10 (90.076757, 12) -> (89.85608, 11.942432)
  line L11 (89.85608, 11.942432) -> (90, 12)
  line L12 (90, 12) -> (60, 12)
  line L13 (60, 12) -> (60.14392, 11.942432)
  line L14 (102, 9.933067) -> (102, 0)
  line L15 (102, 0) -> (140.076757, 0)
  line L16 (140.076757, 0) -> (102, 9.933067)
  line L17 (109.923243, 12) -> (148, 2.066933)
  line L18 (148, 2.066933) -> (148, 12)
  line L19 (148, 12) -> (109.923243, 12)
  line L20 (152, 9.933067) -> (152, 0)
  line L21 (152, 0) -> (190.076757, 0)
  line L22 (190.076757, 0) -> (152, 9.933067)
  line L23 (159.923243, 12) -> (198, 2.066933)
  line L24 (198, 2.066933) -> (198, 12)
  line L25 (198, 12) -> (159.923243, 12)
  line L26 (240.076757, 0) -> (202, 9.933067)
  line L27 (202, 9.933067) -> (202, 0)
  line L28 (202, 0) -> (240.076757, 0)
  line L29 (209.923243, 12) -> (248, 2.066933)
  line L30 (248, 2.066933) -> (248, 12)
  line L31 (248, 12) -> (209.923243, 12)
  line L32 (252, 2.066933) -> (290.076757, 12)
  line L33 (290.076757, 12) -> (252, 12)
  line L34 (252, 12) -> (252, 2.066933)
  line L35 (259.923243, 0) -> (298, 0)
  line L36 (298, 0) -> (298, 9.933067)
  line L37 (298, 9.933067) -> (259.923243, 0)
  line L38 (302, 2.066933) -> (340.076757, 12)
  line L39 (340.076757, 12) -> (302, 12)
  line L40 (302, 12) -> (302, 2.066933)
  line L41 (309.923243, 0) -> (348, 0)
  line L42 (348, 0) -> (348, 9.933067)
  line L43 (348, 9.933067) -> (309.923243, 0)
  line L44 (352, 2.066933) -> (390.076757, 12)
  line L45 (390.076757, 12) -> (352, 12)
  line L46 (352, 12) -> (352, 2.066933)
  line L47 (359.923243, 0) -> (398, 0)
  line L48 (398, 0) -> (398, 9.933067)
  line L49 (398, 9.933067) -> (359.923243, 0)
  line L50 (402, 2.066933) -> (440.076757, 12)
  line L51 (440.076757, 12) -> (402, 12)
  line L52 (402, 12) -> (402, 2.066933)
  line L53 (409.923243, 0) -> (448, 0)
  line L54 (448, 0) -> (448, 9.933067)
  line L55 (448, 9.933067) -> (409.923243, 0)
extrude "押し出し17" cut sketch "SCfront outline for 押し出し17" against normal through all
sketch "スケッチ11" plane through (-202, -25, 10) normal (-1, 0, 0) x (0, 0, 1)
  line L0 (12, 4) -> (0, 4)
  line L1 (0, 0) -> (0, 4)
  line L2 (0, 0) -> (16, 0)
  line L3 (16, 0) -> (16, 50)
  line L4 (16, 50) -> (0, 50)
  line L5 (0, 46) -> (0, 50)
  line L6 (0, 46) -> (12, 46)
  line L7 (12, 46) -> (12, 4)
  line L8 (-13.919969, 46) -> (-6.080031, 46)
  line L9 (-6.080031, 46) -> (-10, 32.28011)
  line L10 (-10, 32.28011) -> (-13.919969, 46)
  line L11 (-16, 38.71989) -> (-12.080031, 25)
  line L12 (-12.080031, 25) -> (-16, 11.28011)
  line L13 (-16, 11.28011) -> (-16, 38.71989)
  line L14 (-13.919969, 4) -> (-10, 17.71989)
  line L15 (-10, 17.71989) -> (-6.080031, 4)
  line L16 (-6.080031, 4) -> (-13.919969, 4)
  line L17 (-4, 11.28011) -> (-7.919969, 25)
  line L18 (-7.919969, 25) -> (-4, 38.71989)
  line L19 (-4, 38.71989) -> (-4, 11.28011)
  line L20 (-20, 0) -> (0, 0)
  line L21 (0, 0) -> (0, 50)
  line L22 (0, 50) -> (-20, 50)
  line L23 (-20, 50) -> (-20, 0)
  line L24 (12, 38.71989) -> (2.080031, 4)
  line L25 (9.919969, 46) -> (0, 11.28011)
  line L26 (2.080031, 46) -> (12, 11.28011)
  line L27 (0, 38.71989) -> (9.919969, 4)
  point P0 (-10, 25)
  point P1 (6, 25)
  point P2 (16, 4)
  point P3 (6, 17.71989)
  point P4 (8.080031, 25)
  point P5 (-4, 0)
  point P6 (3.919969, 25)
  point P7 (6, 32.28011)
  point P8 (16, 50)
  point P9 (16, 46)
  point P10 (16, 50)
  point P11 (-4, 50)
  point P12 (16, 0)
  point P13 (16, 0)
  point P14 (8.080031, 25)
  point P15 (12, 38.71989)
  point P16 (6, 32.28011)
  point P17 (2.080031, 46)
  point P18 (0, 38.71989)
  point P19 (3.919969, 25)
  point P20 (0, 4)
  point P21 (2.080031, 4)
  point P22 (6, 17.71989)
  point P23 (9.919969, 4)
  dimension "d125" = 16
  constraints: 8 end point, 1 horizontal, 21 other
  measures "d125" distance of point (-10, 25) point (6, 25)
sketch "スケッチ11 outline for 押し出し18" plane through (-202, -25, 10) normal (-1, 0, 0) x (0, 0, 1)
  line L0 (8.080031, 25) -> (12, 38.71989)
  line L1 (12, 11.28011) -> (8.080031, 25)
  line L2 (12, 4) -> (12, 11.28011)
  line L3 (9.919969, 4) -> (12, 4)
  line L4 (6, 17.71989) -> (9.919969, 4)
  line L5 (2.080031, 4) -> (6, 17.71989)
  line L6 (0, 4) -> (2.080031, 4)
  line L7 (0, 11.28011) -> (0, 4)
  line L8 (3.919969, 25) -> (0, 11.28011)
  line L9 (0, 38.71989) -> (3.919969, 25)
  line L10 (0, 46) -> (0, 38.71989)
  line L11 (2.080031, 46) -> (0, 46)
  line L12 (6, 32.28011) -> (2.080031, 46)
  line L13 (9.919969, 46) -> (6, 32.28011)
  line L14 (12, 46) -> (9.919969, 46)
  line L15 (12, 38.71989) -> (12, 46)
extrude "押し出し18" add sketch "スケッチ11 outline for 押し出し18" against normal blind 4
mirror "ミラー3" about plane through (0, 0, 0) normal (1, 0, 0) of "押し出し18"